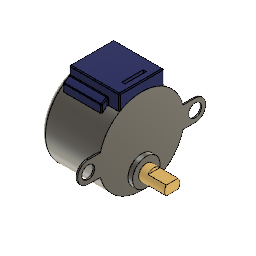
Stepper_Motor_28BYJ-48_v2 (Autodesk Fusion 360 design; units mm, degrees)
Autodesk Fusion 360 part; units mm, degrees
sketch "Layout" plane through (0, 0, 0) normal (1, 0, 0) x (0, 1, 0)
  circle A0 centre (0, 0) radius 14
  circle A1 centre (-17.5, 0) radius 2.1
  line L0 (-29.5, 0) -> (0, 0) construction
  line L1 (-7.3, 17) -> (7.3, 17)
  line L2 (0, 1.75) -> (0, 22.5) construction
  line L3 (-7.3, 17) -> (-7.3, 11.9461)
  line L4 (-13.5554, 3.5) -> (-17.5, 3.5)
  arc A2 (-17.5, 3.5) -> (-17.5, -3.5) centre (-17.5, 0) ccw
  line L5 (-17.5, -3.5) -> (-13.5554, -3.5)
  line L6 (13.5554, 3.5) -> (17.5, 3.5)
  line L7 (17.5, -3.5) -> (13.5554, -3.5)
  arc A3 (17.5, -3.5) -> (17.5, 3.5) centre (17.5, 0) ccw
  circle A4 centre (17.5, 0) radius 2.1
  line L8 (7.3, 17) -> (7.3, 11.9461)
  circle A5 centre (0, -8) radius 4.5
  circle A6 centre (0, -8) radius 2.5
  line L9 (-1.9615, -6.45) -> (1.9615, -6.45)
  line L10 (-1.9615, -9.55) -> (1.9615, -9.55)
  arc A7 (-7.2055, 14.2857) -> (-9.3, 13.0196) centre (0, 0) ccw
  line L11 (-9.3, 13.0196) -> (-9.3, 10.4647)
  line L12 (9.3, 13.0196) -> (9.3, 10.4647)
  arc A8 (9.3, 13.0196) -> (7.2055, 14.2857) centre (0, 0) ccw
  point P0 (0, 17)
  dimension "d1" = 28
  dimension "d2" = 4.2
  dimension "d3" = 17.5
  dimension "d4" = 14.6
  dimension "d5" = 17
  dimension "d6" = 3.5
  dimension "d8" = 9
  dimension "d9" = 5
  dimension "d10" = 1.55
  dimension "d11" = 1.55
  dimension "d12" = 8
  dimension "d13" = 2
  dimension "d14" = 2
  constraint coincident A0.centre L0.end
  constraint horizontal L0
  constraint coincident A1.centre L0
  constraint horizontal L1
  constraint midpoint L1 P0
  constraint coincident P0 L2
  constraint coincident A0 L3.end
  constraint perpendicular L1 L3
  constraint coincident A0 L4.start
  constraint horizontal L4
  constraint vertical A1.centre L4.end
  constraint coincident A1.centre A2.centre
  constraint coincident A0 L5.end
  constraint tangent A2 L5
  constraint horizontal L5
  constraint symmetric A1 L2 A4
  constraint symmetric L1.start L2 L1.end
  constraint symmetric L2 L3.end L8.end
  constraint symmetric L2 L4.start L6.start
  constraint symmetric L2 L4.end L6.end
  constraint symmetric L2 A2.end L7.start
  constraint symmetric L2 A2 A3
  constraint symmetric L2 L5.end L7.end
  constraint coincident L2 A5.centre
  constraint concentric A5 A6
  constraint coincident A6 L9.start
  constraint coincident A6 L9.end
  constraint horizontal L9
  constraint coincident A6 L10.start
  constraint coincident A6 L10.end
  constraint horizontal L10
  constraint coincident A0 L11.end
  constraint vertical L11
  constraint symmetric L2 A7.start A8.end
  constraint symmetric L2 A7.end L12.start
  constraint symmetric L2 A7 A8
  constraint symmetric L2 L11.end L12.end
  measures "d1" diameter of A0
  measures "d2" diameter of A1
  measures "d3" distance of A0.centre A1.centre
  measures "d4" distance of L1.start L1.end
  measures "d5" distance of A0.centre L1
  measures "d6" radius of A2
  measures "d8" diameter of A5
  measures "d9" diameter of A6
  measures "d10" distance of A5.centre L9
  measures "d11" distance of A5.centre L10
  measures "d12" distance of A0.centre A5.centre
  measures "d13" distance of A0 A7
  measures "d14" distance of L3 L11
extrude "Extrude1" add sketch "Layout" against normal blind 19 contours A0 | A5 | A6 L9 L10 | A6 L9 | A6 L10 makes body 1
extrude "Extrude2" add sketch "Layout" against normal blind 0.5 contours A0 L6 L7 A3 | A0 L4 A2 L5 bodies 1
extrude "Extrude3" add sketch "Layout" along normal blind 1.5 contours A5 bodies 1
extrude "Extrude4" add sketch "Layout" along normal blind 10 separate body contours A6 L9 L10 makes body 2
extrude "Extrude5" add sketch "Layout" along normal blind 4 contours A6 L9 | A6 L10 bodies 2
extrude "Extrude6" add sketch "Layout" against normal blind 16.5 separate body contours A0 L8 L12 A8 | A0 L1 L3 L8 | A0 L3 A7 L11 makes body 3
extrude "Extrude7" cut sketch "Layout" against normal blind 3.8 contours A0 L8 L12 A8 | A0 L3 A7 L11 bodies 3
sketch "Wire Entry" plane through (0, 0, 17) normal (0, 0, 1) x (-1, 0, 0)
  line L0 (0, 7.3) -> (0, -7.3)
  line L1 (0, -7.3) -> (16.5, -7.3)
  line L2 (16.5, -7.3) -> (16.5, 7.3)
  line L3 (16.5, 7.3) -> (0, 7.3)
  line L4 (3, -3.5) -> (2, -3.5)
  line L5 (2, -3.5) -> (2, 3.5)
  line L6 (2, 3.5) -> (3, 3.5)
  line L7 (3, 3.5) -> (3, -3.5)
  line L8 (0, 7.3) -> (0, -7.3)
  line L9 (-1.75, 0) -> (-22.5, 0)
  point P0 (2, 0)
  dimension "d29" = 7
  dimension "d30" = 1
  dimension "d31" = 2
  constraint horizontal L4
  constraint vertical L5
  constraint horizontal L6
  constraint vertical L7
  constraint midpoint L5 P0
  constraint coincident P0 L9
  measures "d29" distance of L4.start L6.end
  measures "d30" distance of L5.end L6.end
  measures "d31" distance of L5 L8
extrude "Extrude8" cut sketch "Wire Entry" along normal up to surface contours L4 L5 L6 L7 end surface at (-12.6667, 0, 14) on bodies 1 bodies 3
fillet "Fillet1" radius 0.3 22 edges at (-8.25, 7.3, 17) (0, 7.3, 14.4731) (0, 0, 17) (0, -7.3, 14.4731) (-8.25, -7.3, 17) (-16.5, 0, 17) (-10.15, 9.3, 13.0196) (-3.8, 8.3223, 13.6653) (-16.5, 8.3223, 13.6653) (-3.8, 9.3, 11.7422) (-16.5, 9.3, 11.7422) (-3.8, 7.3, 13.0919) (-10.15, 7.3, 14.2376) (-16.5, 7.3, 15.6188) (-16.5, -7.3, 15.6188) (-16.5, -8.3223, 13.6653) (-16.5, -9.3, 11.7422) (-10.15, -9.3, 13.0196) (-10.15, -7.3, 14.2376) (-3.8, -8.3223, 13.6653) (-3.8, -9.3, 11.7422) (-3.8, -7.3, 13.0919) on bodies 3
fillet "Fillet2" radius 1.5 1 edges at (-19, -13.0526, 5.0626) on bodies 1
copy_body "CopyPasteBodies1" bodies 1 3 2 makes body 4 makes body 5 makes body 6 in component "Motor Assembly"
component "Motor Assembly" placed x (1, 0, 0) y (0, 1, 0) z (0, 0, 1) at (0, 0, 0)
equation "d3 = ( 35 / 2 ) * 1 mm"
equation "d10 = ( 3.1 / 2 ) * 1 mm"
equation "d11 = d10"
named bodies: "Motor Body", "Shaft", "Cap"
